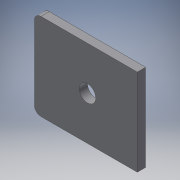
# Autodesk Inventor part: Wiper nut holder
Saved by Autodesk Inventor 2019 (Build 230136000, 136)
## iProperties
Created: 2020-03-14
Part Number: Wiper nut holder
Material: Generic
Document SubType Name: Modeling
Designer: Vijay
Density: 1 g/cm^3
Appearance: Default
Author: Vijay
Autodesk Inventor part; units mm, degrees
ref_plane "YZ Plane" through (0, 0, 0) normal (1, 0, 0) x (0, 1, 0)
ref_plane "XZ Plane" through (0, 0, 0) normal (0, 1, 0) x (-1, 0, 0)
ref_plane "XY Plane" through (0, 0, 0) normal (0, 0, 1) x (1, 0, 0)
sketch "Sketch1" plane through (0, 0, 0) normal (0, 0, 1) x (1, 0, 0)
  line L0 (-49.5875, 0) -> (0, 0)
  line L1 (0, 0) -> (0, -41.788)
  line L2 (0, -41.788) -> (-49.5875, -41.788)
  line L3 (-49.5875, -41.788) -> (-49.5875, 0)
  circle A0 centre (-24, -20.894) radius 3.4749 projected
  circle A1 centre (-24, -20.894) radius 4
  point P0 (0, 0)
  dimension "d0" = 8
  constraints: 8 end point, 2 parallel, 1 centre point, 1 coincident, 1 horizontal, 1 perpendicular, 2 other
  measures "d0" diameter of A1
extrude "Extrusion1" add sketch "Sketch1" along normal blind 4 contours L0 L1 L2 L3
fillet "Fillet1" radius 3.175 2 edges at (-49.5875, 0, 2) (-49.5875, -41.788, 2)
sketch "Sketch2" plane through (0, 0, 4) normal (0, 0, 1) x (1, 0, 0)
  line L0 (-42.7117, -37.788) -> (-36.7117, -37.788) construction
  line L1 (-42.7117, -37.788) -> (-42.7117, -41.788) construction
  line L2 (-36.7117, -41.788) -> (-42.7117, -41.788) construction
  line L3 (-36.7117, -37.788) -> (-36.7117, -41.788) construction
  line L4 (-21.5117, -37.788) -> (-15.5117, -37.788) construction
  line L5 (-21.5117, -37.788) -> (-21.5117, -41.788) construction
  line L6 (-15.5117, -41.788) -> (-21.5117, -41.788) construction
  line L7 (-15.5117, -37.788) -> (-15.5117, -41.788) construction
  line L8 (-21.5117, 0) -> (-15.5117, 0) construction
  line L9 (-21.5117, 0) -> (-21.5117, -4) construction
  line L10 (-15.5117, -4) -> (-21.5117, -4) construction
  line L11 (-15.5117, 0) -> (-15.5117, -4) construction
  line L12 (-42.7117, 0) -> (-36.7117, 0) construction
  line L13 (-42.7117, 0) -> (-42.7117, -4) construction
  line L14 (-36.7117, -4) -> (-42.7117, -4) construction
  line L15 (-36.7117, 0) -> (-36.7117, -4) construction
  line L16 (-27.4117, -4) -> (-30.8117, -4) construction
  line L17 (-27.4117, 0) -> (-27.4117, -4) construction
  line L18 (-30.8117, 0) -> (-27.4117, 0) construction
  line L19 (-30.8117, 0) -> (-30.8117, -4) construction
  line L20 (-27.4117, -41.788) -> (-30.8117, -41.788) construction
  line L21 (-27.4117, -37.788) -> (-27.4117, -41.788) construction
  line L22 (-30.8117, -37.788) -> (-27.4117, -37.788) construction
  line L23 (-30.8117, -37.788) -> (-30.8117, -41.788) construction
  line L24 (-42.9117, -41.988) -> (-42.9117, -37.588)
  line L25 (-42.9117, -37.588) -> (-36.5117, -37.588)
  line L26 (-36.5117, -37.588) -> (-36.5117, -41.988)
  line L27 (-36.5117, -41.988) -> (-42.9117, -41.988)
  line L28 (-21.7117, -41.988) -> (-21.7117, -37.588)
  line L29 (-21.7117, -37.588) -> (-15.3117, -37.588)
  line L30 (-15.3117, -37.588) -> (-15.3117, -41.988)
  line L31 (-15.3117, -41.988) -> (-21.7117, -41.988)
  line L32 (-42.9117, -4.2) -> (-42.9117, 0.2)
  line L33 (-42.9117, 0.2) -> (-36.5117, 0.2)
  line L34 (-36.5117, 0.2) -> (-36.5117, -4.2)
  line L35 (-36.5117, -4.2) -> (-42.9117, -4.2)
  line L36 (-21.7117, -4.2) -> (-21.7117, 0.2)
  line L37 (-21.7117, 0.2) -> (-15.3117, 0.2)
  line L38 (-15.3117, 0.2) -> (-15.3117, -4.2)
  line L39 (-15.3117, -4.2) -> (-21.7117, -4.2)
  circle A0 centre (-29.1117, -39.788) radius 1.6
  circle A1 centre (-29.1117, -2) radius 1.6
  point P0 (0, 0)
  dimension "d4" = 0.2
  dimension "d5" = 0.2
  dimension "d6" = 0.2
  dimension "d7" = 0.2
  dimension "d8" = 3.2
  dimension "d9" = 3.2
  constraints: 32 end point, 2 centre point, 12 other
  measures "d4" distance between parallel lines of L1 L24
  measures "d5" distance between parallel lines of L5 L28
  measures "d6" distance between parallel lines of L13 L32
  measures "d7" distance between parallel lines of L9 L36
  measures "d8" diameter of A0
  measures "d9" diameter of A1
extrude "Extrusion2" cut sketch "Sketch2" against normal blind 4
body "Solid1"
